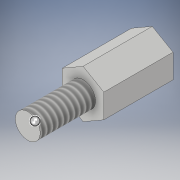
# Autodesk Inventor part: Spacer-M2-05
Saved by Autodesk Inventor 2019 (Build 230136000, 136)
## iProperties
Created: 2018-04-28
Part Number: Spacer-M2-05
Material: Generic
Document SubType Name: Modeling
Designer: Fierl
Density: 1 g/cm^3
Appearance: Default
length: 20
Author: Fierl
Autodesk Inventor part; units mm, degrees
ref_plane "YZ Plane" through (0, 0, 0) normal (1, 0, 0) x (0, 1, 0)
ref_plane "XZ Plane" through (0, 0, 0) normal (0, 1, 0) x (-1, 0, 0)
ref_plane "XY Plane" through (0, 0, 0) normal (0, 0, 1) x (1, 0, 0)
sketch "Sketch1" plane through (0, 0, 0) normal (0, 0, 1) x (1, 0, 0)
  line L0 (1.5, 0.866) -> (1.5, -0.866)
  line L1 (1.5, -0.866) -> (0, -1.732)
  line L2 (0, -1.732) -> (-1.5, -0.866)
  line L3 (-1.5, 0.866) -> (-1.5, -0.866)
  line L4 (-1.5, 0.866) -> (0, 1.732)
  line L5 (0, 1.732) -> (1.5, 0.866)
  circle A0 centre (0, 0) radius 1.732 construction
  line L6 (0, 30.018) -> (0, -6.2677) construction
  line L7 (0, -13.5249) -> (0, 37.2751) projected
  line L8 (-2.4248, 0) -> (2.4248, 0) projected
  dimension "d0" = 3.464
  dimension "d20" = 2.9999
  dimension "d21" = 1.732
  constraints: 14 end point, 6 point on circle, 3 coincident, 3 equal length, 2 parallel, 2 point on line, 1 centre point, 1 vertical
  measures "d0" diameter of A0
  measures "d20" distance between parallel lines of L0 L3
  measures "d21" distance of L0.start L0.end
extrude "Hexagon1" add sketch "Sketch1" along normal blind 5
hole "Hole1" at (0, 0, 0) direction (0, 0, 1) diameter 1.567 depth 4 thread size "M2x0.4" class "6H" standard "ISO Metric profile"
sketch "Sketch2" plane through (0, 0, 5) normal (0, 0, 1) x (1, 0, 0)
  circle A0 centre (0, 0) radius 0.9
  dimension "d22" = 1.8
  constraints: 1 centre point, 1 coincident
  measures "d22" diameter of A0
extrude "Extrusion2" add sketch "Sketch2" along normal blind 4
thread "Thread3" size "M2x0.4" class "6g" standard "ISO Metric profile" full length
body "Solid1"
